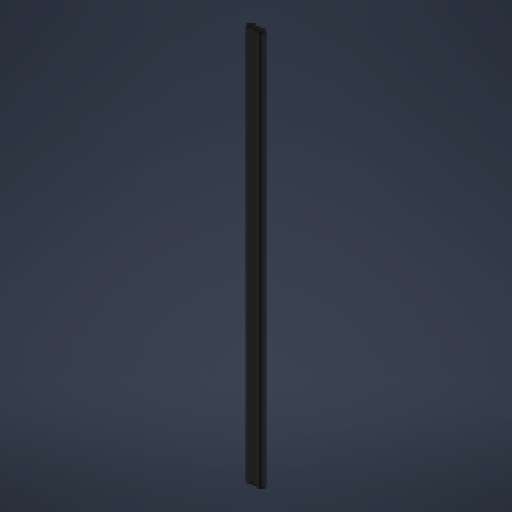
# Autodesk Inventor part: 3DPRINT,BACK,RAIL
Saved by Autodesk Inventor 2026.1 (Build 301233020, 233B)
## iProperties
Created: 2026-04-01
Part Number: 3DPRINT,BACK,RAIL
Material: ABS Plastic
Document SubType Name: Modeling
Designer: Owen L
Density: 1.06 g/cm^3
Appearance: Smooth - Black
Author: Owen L
Autodesk Inventor part; units mm, degrees
ref_plane "YZ Plane" through (0, 0, 0) normal (1, 0, 0) x (0, 1, 0)
ref_plane "XZ Plane" through (0, 0, 0) normal (0, 1, 0) x (-1, 0, 0)
ref_plane "XY Plane" through (0, 0, 0) normal (0, 0, 1) x (1, 0, 0)
sketch "Sketch1" plane through (0, 0, 0) normal (1, 0, 0) x (0, 1, 0)
  line L0 (-177.8, 6.35) -> (177.8, 6.35)
  line L1 (177.8, 6.35) -> (177.8, -6.35)
  line L2 (177.8, -6.35) -> (-177.8, -6.35)
  line L3 (-177.8, -6.35) -> (-177.8, 6.35)
  line L4 (-177.8, 6.35) -> (177.8, -6.35) construction
  line L5 (177.8, 6.35) -> (-177.8, -6.35) construction
  point P0 (0, 0)
  dimension "d0" = 355.6
  dimension "d1" = 12.7
  constraints: 12 end point, 2 midpoint, 2 parallel, 1 horizontal, 1 perpendicular
  measures "d0" distance of L1.end L2.end
  measures "d1" distance of L0.end L1.end
extrude "Extrusion1" add sketch "Sketch1" along normal blind 12.7
sketch "Sketch2" plane through (0, -177.8, -6.35) normal (0, -1, 0) x (1, 0, 0)
  circle A0 centre (6.35, 79.518) radius 76.2
  line L0 (0, 0) -> (12.7, 0) projected
  point P0 (0, 6.35)
  point P1 (6.35, 3.318)
  point P2 (6.35, 0)
  point P3 (6.35, 0)
  point P4 (6.35, 0)
  dimension "d4" = 152.4
  dimension "d5" = 3.318
  constraints: 3 midpoint, 3 vertical alignment, 2 other
  measures "d5" distance of point (6.35, 0) point (6.35, 3.318)
extrude "Extrusion2" cut sketch "Sketch2" against normal through all
body "Solid1"
